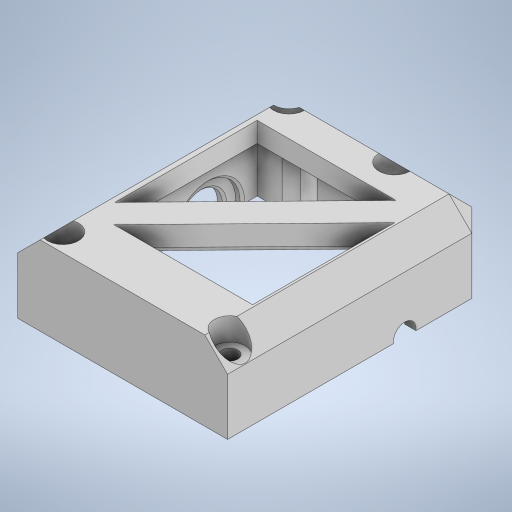
# Autodesk Inventor part: Arm_1_b
Saved by Autodesk Inventor 2023 (Build 270158000, 158)
## iProperties
Created: 2025-02-10
Part Number: Arm_1_b
Material: Generic
Document SubType Name: Modeling
Designer: Swoby
Density: 1 g/cm^3
Appearance: Default
Author: Swoby
Autodesk Inventor part; units mm, degrees
sketch "Sketch1" plane through (0, 0, 0) normal (0, 1, 0) x (-1, 0, 0)
  line L0 (0, 0) -> (3.1, 0)
  line L1 (0, 0) -> (0, -7.4)
  line L2 (0, -7.4) -> (1.5, -7.4)
  line L3 (1.5, -7.4) -> (1.5, -5)
  line L4 (1.5, -5) -> (3.1, -5)
  line L5 (3.1, -5) -> (3.1, 0)
  line L6 (0, -7.4) -> (0, -10.65)
  line L7 (0, -10.65) -> (-7.5, -10.65)
  line L8 (-7.5, -10.65) -> (-7.5, -17.75)
  line L9 (-7.5, -17.75) -> (-11.2, -17.75)
  line L10 (-11.2, -17.75) -> (-11.2, -10.65)
  line L11 (-11.2, -10.65) -> (-31.3, -10.65)
  line L12 (-31.3, -10.65) -> (-31.3, -19.75)
  line L13 (-31.3, -19.75) -> (-36.7, -19.75)
  line L14 (-36.7, -19.75) -> (-36.7, -10.65)
  line L15 (-36.7, -10.65) -> (-40.6, -10.65)
  line L16 (-40.6, -10.65) -> (-40.6, 30.95)
  line L17 (-40.6, 30.95) -> (-11.2, 30.95)
  line L18 (-11.2, 30.95) -> (-11.2, 38.05)
  line L19 (-11.2, 38.05) -> (-7.5, 38.05)
  line L20 (-7.5, 38.05) -> (-7.5, 30.95)
  line L21 (-7.5, 30.95) -> (0, 30.95)
  line L22 (0, 0) -> (0, 30.95)
  line L23 (3.1, 0) -> (3.1, 53.05)
  line L24 (-43.1, -19.75) -> (-43.1, 53.05)
  line L25 (3.1, -5) -> (3.1, -19.75)
  line L26 (3.1, -19.75) -> (-43.1047, -19.75)
  line L27 (-43.1, 53.05) -> (3.1, 53.05) construction
  line L28 (-43.1, 64.5353) -> (3.1, 64.5353) construction
  line L29 (3.1, 64.5353) -> (3.1, 93.4653) construction
  line L30 (3.1, 93.4653) -> (-43.1, 93.4653) construction
  line L31 (-43.1, 93.4653) -> (-43.1, 64.5353)
  line L32 (3.1, 53.05) -> (10.1, 60.05)
  line L33 (10.1, 60.05) -> (10.1, 95.4653)
  line L34 (10.1, 95.4653) -> (4.1, 95.4653)
  line L35 (4.1, 95.4653) -> (4.1, 62.5353)
  line L36 (4.1, 62.5353) -> (-5.3853, 53.05)
  line L37 (-20, 53.05) -> (-20, 57.2324) construction
  line L38 (-43.1, 64.5353) -> (-43.1, 93.4653)
  line L39 (-43.1, 53.05) -> (-50.1, 60.05)
  line L40 (-50.1, 60.05) -> (-50.1, 95.4653)
  line L41 (-50.1, 95.4653) -> (-44.1, 95.4653)
  line L42 (-44.1, 95.4653) -> (-44.1, 62.5353)
  line L43 (-44.1, 62.5353) -> (-34.6147, 53.05)
  line L44 (4.1, 62.5353) -> (10.1, 60.05) construction
  line L45 (-5.3853, 53.05) -> (-34.6147, 53.05)
  line L46 (-44.1, 79.0003) -> (-41.1, 79.0003)
  line L47 (-44.1, 81.3003) -> (-41.1, 81.3003)
  line L48 (-41.1, 81.3003) -> (-41.1, 79.0003)
  line L49 (-44.1, 81.3003) -> (-44.1, 79.0003)
  line L50 (-40.6, -2.5) -> (-40.6, 0)
  line L51 (-40.6, 0) -> (-43.1, 0)
  line L52 (-40.6, -2.5) -> (-43.1, -2.5)
  line L53 (-43.1, 0) -> (-43.1, -2.5)
  point P0 (1.55, 0)
  point P1 (-43.1, 65.1211)
  point P2 (-43.1, 94.8791)
  point P3 (3.1, 79.0003)
  dimension "d1" = 1.5
  dimension "d3" = 1.6
  dimension "d4" = 10
  dimension "d5" = 14.8
  dimension "d6" = 7.5
  dimension "d7" = 3.7
  dimension "d9" = 10.65
  dimension "d10" = 41.6
  dimension "d11" = 40.6
  dimension "d12" = 7.1
  dimension "d13" = 3.9
  dimension "d14" = 5.4
  dimension "d16" = 7.1
  dimension "d17" = 46.2
  dimension "d18" = 2
  dimension "d19" = 15
  dimension "d20" = 28.93
  dimension "d21" = 6
  dimension "d22" = 135
  dimension "d23" = 67.5
  dimension "d24" = 135
  dimension "d26" = 2
  dimension "d27" = 32.93
  dimension "d31" = 79.0003
  dimension "d33" = 1
  dimension "d34" = 3
  dimension "d35" = 2.3
  dimension "d70" = 5
  constraints: 108 end point, 24 perpendicular, 15 point on line, 7 collinear, 7 parallel, 7 vertical, 5 symmetric about line, 4 horizontal, 4 midpoint
  measures "d1" distance of L1.end L2.end
  measures "d3" distance of L3.end L4.end
  measures "d4" diameter of L4 L0
  measures "d5" diameter of L2 L0
  measures "d6" distance of L6.end L7.end
  measures "d7" distance of L8.end L9.end
  measures "d9" distance from line of L7 L0.start
  measures "d10" distance between parallel lines of L7 L21
  measures "d11" distance between parallel lines of L16 L22
  measures "d12" distance of L7.end L8.end
  measures "d13" distance of L14.end L15.end
  measures "d14" distance of L12.end L13.end
  measures "d16" distance of L19.end L20.end
  measures "d17" distance between parallel lines of L24 L23
  measures "d18" distance between parallel lines of L26 L9
  measures "d19" distance from line of L24.end L19
  measures "d20" distance of L28.end L29.end
  measures "d21" distance of L33.end L34.end
  measures "d22" angle of L23 L32
  measures "d23" angle of L32 L44
  measures "d24" angle of L32 L33
  measures "d26" distance from line of L30 L34.end
  measures "d27" distance from line of L34 L35.end
  measures "d31" vertical distance of point (3.1, 79) L0.start
  measures "d33" distance between parallel lines of L29 L35
  measures "d34" distance of L47.start L47.end
  measures "d35" distance of L47.end L46.end
  measures "d70" diameter of L52 L51
extrude "Extrusion1" add sketch "Sketch1" along normal mid plane 34 contours L22 L21 L20 L19 L18 L17 L16 L51 L24 L39 L40 L41 L42 L43 L45 L36 L35 L34 L33 L32 L23 L0 | L0 L5 L4 L3 L2 L1 | L2 L3 L4 L25 L26 L12 L11 L10 L9 L8 L7 L6 | L26 L24 L52 L16 L15 L14 | L24 L51 L16 L52
revolve "Revolution1" cut sketch "Sketch1" angle 360 about axis through (0, 0, 0) along (-1, 0, 0) contours L0 L5 L4 L3 L2 L1 | L24 L51 L16 L52
revolve "Revolution2" add sketch "Sketch1" angle 360 about axis through (44.1, 0, 79.0003) along (-1, 0, 0) contours L42 L47 L31 L46 | L31 L47 L48 L46
sketch "Sketch2" plane through (-4.1, -17, 62.5353) normal (1, 0, 0) x (0, 0, -1)
  line L0 (-32.93, 34) -> (0, 0) construction
  line L1 (0, 34) -> (-32.93, 0) construction
  circle A0 centre (-16.465, 17) radius 3.4
  line L2 (-16.465, 17) -> (-5.3446, 17) construction
  line L3 (-16.465, 17) -> (-3.5603, 29.9047) construction
  line L4 (-16.465, 17) -> (-3.5603, 4.0953) construction
  circle A1 centre (-3.5603, 29.9047) radius 0.5
  arc A2 (-1.9362, 28.7375) -> (-2.1461, 31.3189) centre (-3.5603, 29.9047) ccw
  arc A3 (-2.1461, 2.6811) -> (-1.9362, 5.2625) centre (-3.5603, 4.0953) ccw
  circle A4 centre (-3.5603, 4.0953) radius 0.5
  line L5 (-11.8688, 21.5962) -> (-9.0757, 18.8031) construction
  line L6 (-11.8688, 12.4038) -> (-9.0757, 15.1969) construction
  line L7 (-9.0757, 15.1969) -> (-1.9362, 5.2625)
  line L8 (-9.0757, 18.8031) -> (-1.9362, 28.7375)
  line L9 (-3.5603, 29.9047) -> (-2.1461, 31.3189) construction
  line L10 (-3.5603, 4.0953) -> (-2.1461, 2.6811) construction
  line L11 (-3.5603, 29.9047) -> (-2.1461, 31.3189) construction
  arc A5 (-9.0757, 18.8031) -> (-9.0757, 15.1969) centre (-6.5668, 17) ccw
  arc A6 (-28.2025, 31.5288) -> (-30.7839, 31.3189) centre (-29.3697, 29.9047) ccw
  line L12 (-18.2681, 24.3893) -> (-28.2025, 31.5288)
  arc A7 (-18.2681, 24.3893) -> (-14.6619, 24.3893) centre (-16.465, 26.8982) ccw
  line L13 (-14.6619, 24.3893) -> (-4.7275, 31.5288)
  arc A8 (-2.1461, 31.3189) -> (-4.7275, 31.5288) centre (-3.5603, 29.9047) ccw
  circle A9 centre (-3.5603, 29.9047) radius 0.5
  circle A10 centre (-29.3697, 29.9047) radius 0.5
  arc A11 (-30.9938, 5.2625) -> (-30.7839, 2.6811) centre (-29.3697, 4.0953) ccw
  line L14 (-23.8543, 15.1969) -> (-30.9938, 5.2625)
  arc A12 (-23.8543, 15.1969) -> (-23.8543, 18.8031) centre (-26.3632, 17) ccw
  line L15 (-23.8543, 18.8031) -> (-30.9938, 28.7375)
  arc A13 (-30.7839, 31.3189) -> (-30.9938, 28.7375) centre (-29.3697, 29.9047) ccw
  circle A14 centre (-29.3697, 29.9047) radius 0.5
  circle A15 centre (-29.3697, 4.0953) radius 0.5
  arc A16 (-4.7275, 2.4712) -> (-2.1461, 2.6811) centre (-3.5603, 4.0953) ccw
  line L16 (-14.6619, 9.6107) -> (-4.7275, 2.4712)
  arc A17 (-14.6619, 9.6107) -> (-18.2681, 9.6107) centre (-16.465, 7.1018) ccw
  line L17 (-18.2681, 9.6107) -> (-28.2025, 2.4712)
  arc A18 (-30.7839, 2.6811) -> (-28.2025, 2.4712) centre (-29.3697, 4.0953) ccw
  circle A19 centre (-29.3697, 4.0953) radius 0.5
  circle A20 centre (-3.5603, 4.0953) radius 0.5
  point P0 (62.5353, 17)
  point P1 (-2.1461, 31.3189)
  point P2 (-30.7839, 31.3189)
  point P3 (-30.7839, 2.6811)
  point P4 (-2.1461, 2.6811)
  dimension "d38" = 6.8
  dimension "d39" = 45
  dimension "d40" = 1
  dimension "d41" = 4
  dimension "d42" = 18.25
  dimension "d43" = 18.25
  dimension "d44" = 4
  dimension "d45" = 1
  dimension "d46" = 3.95
  dimension "d47" = 6.5
  dimension "d48" = 3.95
  dimension "d49" = 6.5
  dimension "d52" = 360
  constraints: 36 end point, 24 point on circle, 21 centre point, 10 coincident, 3 point on line, 3 tangent, 2 midpoint, 1 collinear, 1 horizontal, 1 perpendicular, 73 other
  measures "d38" diameter of A0
  measures "d39" angle of L2 L3
  measures "d40" diameter of A1
  measures "d41" diameter of A2
  measures "d42" distance of L3.end point (-16.465, 17)
  measures "d43" distance of L2.start L4.end
  measures "d44" diameter of A3
  measures "d45" diameter of A4
  measures "d46" distance of L5.start L5.end
  measures "d47" distance between parallel lines of L4 L5
  measures "d48" distance of L6.start L6.end
  measures "d49" distance between parallel lines of L3 L6
extrude "Extrusion2" cut sketch "Sketch2" against normal through all contours A0 | A1 | A4 | A10 | A15
extrude "Extrusion3" cut sketch "Sketch2" against normal blind 4
sketch "Sketch3" plane through (0, 17, 0) normal (0, 1, 0) x (1, 0, 0)
  line L0 (43.1, -53.05) -> (43.1, 19.75) projected
  line L1 (43.1, 19.75) -> (36.7, 19.75) projected
  line L2 (36.7, 19.75) -> (36.7, 10.65) projected
  line L3 (36.7, 10.65) -> (40.6, 10.65) projected
  line L4 (40.6, 10.65) -> (40.6, -30.95) projected
  line L5 (40.6, -30.95) -> (11.2, -30.95) projected
  line L6 (11.2, -30.95) -> (11.2, -38.05) projected
  line L7 (11.2, -38.05) -> (7.5, -38.05) projected
  line L8 (7.5, -38.05) -> (7.5, -30.95) projected
  line L9 (7.5, -30.95) -> (0, -30.95) projected
  line L10 (0, -30.95) -> (0, 10.65) projected
  line L11 (0, 10.65) -> (7.5, 10.65) projected
  line L12 (7.5, 10.65) -> (7.5, 17.75) projected
  line L13 (7.5, 17.75) -> (11.2, 17.75) projected
  line L14 (11.2, 17.75) -> (11.2, 10.65) projected
  line L15 (11.2, 10.65) -> (31.3, 10.65) projected
  line L16 (31.3, 10.65) -> (31.3, 19.75) projected
  line L17 (31.3, 19.75) -> (-3.1, 19.75) projected
  line L18 (-3.1, 19.75) -> (-3.1, -53.05) projected
  line L19 (-3.1, -53.05) -> (-10.1, -60.05) projected
  line L20 (-10.1, -60.05) -> (-10.1, -95.4653) projected
  line L21 (-10.1, -95.4653) -> (-4.1, -95.4653) projected
  line L22 (-4.1, -95.4653) -> (-4.1, -62.5353) projected
  line L23 (-4.1, -62.5353) -> (5.3853, -53.05) projected
  line L24 (5.3853, -53.05) -> (34.6147, -53.05) projected
  line L25 (34.6147, -53.05) -> (44.1, -62.5353) projected
  line L26 (44.1, -62.5353) -> (44.1, -95.4653) projected
  line L27 (44.1, -95.4653) -> (50.1, -95.4653) projected
  line L28 (50.1, -95.4653) -> (50.1, -60.05) projected
  line L29 (50.1, -60.05) -> (43.1, -53.05) projected
  line L30 (31.3, 19.75) -> (36.7, 19.75)
  point P0 (0, 0)
  constraints: 2 end point, 1 collinear
extrude "Extrusion4" add sketch "Sketch3" against normal blind 6.4 contours L2 L3 L4 L5 L6 L7 L8 L9 L10 L11 L12 L13 L14 L15 L16 L30
mirror "Mirror1" about plane through (0, 0, 0) normal (0, 1, 0) of "Extrusion4"
chamfer "Chamfer1" distance 3 angle 45 4 edges at (47.1, -17, 95.4653) (47.1, 17, 95.4653) (-7.1, -17, 95.4653) (-7.1, 17, 95.4653)
chamfer "Chamfer2" distance 5 angle 45 10 edges at (-3.1, -17, 16.65) (43.1, -17, 16.65) (43.1, 0, -19.75) (20, -17, -19.75) (43.1, 17, 16.65) (20, 17, -19.75) (-3.1, 17, 16.65) (-3.1, 0, -19.75) (20, -17, 53.05) (20, 17, 53.05)
chamfer "Chamfer3" distance 2 angle 45 34 edges at (-6.6, -17, 56.55) (0.6426, -17, 57.7926) (-10.1, -17, 76.2576) (-4.1, -17, 77.5003) (39.3574, -17, 57.7926) (46.6, -17, 56.55) (50.1, -17, 76.2576) (44.1, -17, 77.5003) (50.1, 0, 60.05) (-10.1, 0, 60.05) (-6.6, 17, 56.55) (-10.1, 17, 76.2576) (-10.1, 0, 95.4653) (-10.1, 15.5, 93.9653) (-10.1, -15.5, 93.9653) (-4.1, -15.5, 93.9653) (-4.1, 0, 95.4653) (-4.1, 15.5, 93.9653) (-4.1, 17, 77.5003) (0.6426, 17, 57.7926) (39.3574, 17, 57.7926) (46.6, 17, 56.55) (44.1, 17, 77.5003) (50.1, 17, 76.2576) (44.1, 15.5, 93.9653) (44.1, 0, 95.4653) (44.1, -15.5, 93.9653) (50.1, -15.5, 93.9653) (50.1, 0, 95.4653) (50.1, 15.5, 93.9653) (20, -12, 53.05) (20, -17, 48.05) (20, 12, 53.05) (20, 17, 48.05)
sketch "Sketch4" plane through (0, 17, 0) normal (0, 1, 0) x (1, 0, 0)
  line L0 (11.2, 10.65) -> (31.3, 10.65) projected
  line L1 (11.2, 17.75) -> (11.2, 10.65) projected
  line L2 (7.5, 17.75) -> (11.2, 17.75) projected
  line L3 (7.5, 10.65) -> (7.5, 17.75) projected
  line L4 (0, 10.65) -> (7.5, 10.65) projected
  line L5 (0, -30.95) -> (0, 10.65) projected
  line L6 (7.5, -30.95) -> (0, -30.95) projected
  line L7 (7.5, -38.05) -> (7.5, -30.95) projected
  line L8 (11.2, -38.05) -> (7.5, -38.05) projected
  line L9 (11.2, -30.95) -> (11.2, -38.05) projected
  line L10 (40.6, -30.95) -> (11.2, -30.95) projected
  line L11 (40.6, 10.65) -> (40.6, -30.95) projected
  line L12 (36.7, 10.65) -> (40.6, 10.65) projected
  line L13 (36.7, 19.75) -> (36.7, 10.65) projected
  line L14 (31.3, 19.75) -> (36.7, 19.75) projected
  line L15 (31.3, 10.65) -> (31.3, 19.75) projected
  line L16 (33.4802, 7.65) -> (3, 7.65)
  line L17 (7.1198, -27.95) -> (37.6, -27.95)
  line L18 (40.6, 10.65) -> (0, -30.95) construction
  line L19 (33.4802, 7.65) -> (3, -23.5809)
  line L20 (7.1198, -27.95) -> (37.6, 3.2809)
  line L21 (37.6, -27.95) -> (37.6, 3.2809)
  line L22 (37.6, 7.5761) -> (37.6, 7.65)
  line L23 (3, 7.65) -> (3, -23.5809)
  line L24 (3, -27.8761) -> (3, -27.95)
  point P0 (0, 0)
  point P1 (20.3, -10.15)
  dimension "d72" = 3
  dimension "d74" = 3
  dimension "d75" = 3
  dimension "d76" = 3
  dimension "d77" = 3
  dimension "d78" = 3
  constraints: 18 end point, 7 parallel, 2 perpendicular, 2 point on line, 1 horizontal, 1 midpoint
  measures "d72" distance between parallel lines of L10 L17
  measures "d74" distance between parallel lines of L0 L16
  measures "d75" distance from line of point (20.3, -10.15) L19
  measures "d76" distance between parallel lines of L20 L18
  measures "d77" distance between parallel lines of L5 L23
  measures "d78" distance between parallel lines of L11 L21
extrude "Extrusion5" cut sketch "Sketch4" against normal through all contours L19 L23 L16 | L20 L21 L17
chamfer "Chamfer4" distance 2 angle 45 16 edges at (18.2401, -10.6, 7.9655) (22.3599, -10.6, 12.3345) (18.2401, 10.6, 7.9655) (22.3599, 10.6, 12.3345) (18.2401, -10.6, -7.65) (3, -10.6, 7.9655) (3, 10.6, 7.9655) (18.2401, 10.6, -7.65) (37.6, 10.6, 12.3345) (22.3599, 10.6, 27.95) (22.3599, -10.6, 27.95) (37.6, -10.6, 12.3345) (7.5, 0, 30.95) (11.2, 0, 30.95) (7.5, 0, -10.65) (11.2, 0, -10.65)
ref_plane "Work Plane2" through (0, -0.4, 0) normal (0, -1, 0) x (1, 0, 0)
ref_plane "Work Plane3" through (40.6, -10.6, 38.95) normal (0, 0, -1) x (-1, 0, 0)
sketch "Sketch5" plane through (0, -0.4, 0) normal (0, -1, 0) x (1, 0, 0)
  line L0 (62.14, 38.95) -> (-22.14, 38.95) projected
  line L1 (43.1, -14.75) -> (43.1, 53.05) projected
  line L2 (43.1, -14.75) -> (38.1, -19.75) projected
  line L3 (1.9, -19.75) -> (38.1, -19.75) projected
  line L4 (36.7, -19.75) -> (36.7, -10.65) projected
  line L5 (36.7, -10.65) -> (40.6, -10.65) projected
  line L6 (40.6, -10.65) -> (40.6, 30.95) projected
  line L7 (40.6, 30.95) -> (13.2, 30.95) projected
  line L8 (13.2, 30.95) -> (11.2, 32.95) projected
  line L9 (11.2, 32.95) -> (11.2, 38.05) projected
  line L10 (11.2, 38.05) -> (7.5, 38.05) projected
  line L11 (7.5, 38.05) -> (7.5, 32.95) projected
  line L12 (7.5, 32.95) -> (5.5, 30.95) projected
  line L13 (5.5, 30.95) -> (0, 30.95) projected
  line L14 (0, 30.95) -> (0, -10.65) projected
  line L15 (0, -10.65) -> (5.5, -10.65) projected
  line L16 (5.5, -10.65) -> (7.5, -12.65) projected
  line L17 (7.5, -12.65) -> (7.5, -17.75) projected
  line L18 (7.5, -17.75) -> (11.2, -17.75) projected
  line L19 (11.2, -17.75) -> (11.2, -12.65) projected
  line L20 (1, 28.4936) -> (38.2267, -9.65) projected
  line L21 (1, -9.65) -> (1, 28.4936) projected
  line L22 (38.2267, -9.65) -> (1, -9.65) projected
  line L23 (11.2, -12.65) -> (13.2, -10.65) projected
  line L24 (11.2, -17.75) -> (11.2, -12.65) projected
  line L25 (7.5, -17.75) -> (11.2, -17.75) projected
  line L26 (7.5, -12.65) -> (7.5, -17.75) projected
  line L27 (5.5, -10.65) -> (7.5, -12.65) projected
  line L28 (0, -10.65) -> (5.5, -10.65) projected
  line L29 (0, 30.95) -> (0, -10.65) projected
  line L30 (5.5, 30.95) -> (0, 30.95) projected
  line L31 (7.5, 32.95) -> (5.5, 30.95) projected
  line L32 (7.5, 38.05) -> (7.5, 32.95) projected
  line L33 (11.2, 38.05) -> (7.5, 38.05) projected
  line L34 (11.2, 32.95) -> (11.2, 38.05) projected
  line L35 (13.2, 30.95) -> (11.2, 32.95) projected
  line L36 (40.6, 30.95) -> (13.2, 30.95) projected
  line L37 (40.6, -10.65) -> (40.6, 30.95) projected
  line L38 (36.7, -10.65) -> (40.6, -10.65) projected
  line L39 (36.7, -19.75) -> (36.7, -10.65) projected
  line L40 (31.3, -19.75) -> (36.7, -19.75) projected
  line L41 (31.3, -10.65) -> (31.3, -19.75) projected
  line L42 (13.2, -10.65) -> (31.3, -10.65) projected
  line L43 (39.6, -8.1936) -> (2.3733, 29.95) projected
  line L44 (39.6, 29.95) -> (39.6, -8.1936) projected
  line L45 (2.3733, 29.95) -> (39.6, 29.95) projected
  line L46 (1.9, -19.75) -> (-3.1, -14.75) projected
  line L47 (-3.1, 53.05) -> (-3.1, -14.75) projected
  circle A0 centre (26.1, -14.75) radius 2.15
  line L48 (36.7, -14.75) -> (43.1, -14.75) construction
  line L49 (26.1, -14.75) -> (26.1, -19.75) construction
  circle A1 centre (2.9, -14.75) radius 2.15
  circle A2 centre (39.6, 34.95) radius 2.15
  circle A3 centre (2.9, 34.95) radius 2.15
  circle A4 centre (2.9, -14.75) radius 1.75
  circle A5 centre (26.1, -14.75) radius 1.75
  circle A6 centre (39.6, 34.95) radius 1.75
  circle A7 centre (2.9, 34.95) radius 1.75
  circle A8 centre (26.1, -14.75) radius 3.4
  circle A9 centre (2.9, -14.75) radius 3.4
  circle A10 centre (2.9, 34.95) radius 3.4
  circle A11 centre (39.6, 34.95) radius 3.4
  point P0 (0, 0)
  dimension "d86" = 4.3
  dimension "d87" = 5
  dimension "d89" = 4.3
  dimension "d90" = 6
  dimension "d91" = 4.3
  dimension "d92" = 4
  dimension "d93" = 8
  dimension "d94" = 4.3
  dimension "d95" = 4
  dimension "d96" = 6
  dimension "d101" = 3.5
  dimension "d102" = 3.5
  dimension "d103" = 3.5
  dimension "d104" = 3.5
  dimension "d105" = 6.8
  dimension "d106" = 6.8
  dimension "d107" = 6.8
  dimension "d108" = 6.8
  dimension "d111" = 17
  constraints: 12 centre point, 8 coincident, 6 point on line, 4 end point, 1 perpendicular, 1 vertical
  measures "d86" diameter of A0
  measures "d87" distance between parallel lines of L3 L48
  measures "d89" diameter of A1
  measures "d90" distance from line of L47 A1.centre
  measures "d91" diameter of A2
  measures "d92" distance from line of L0 A2.centre
  measures "d93" distance between parallel lines of L0 L36
  measures "d94" diameter of A3
  measures "d95" distance from line of L0 A3.centre
  measures "d96" distance from line of L47 A3.centre
  measures "d101" diameter of A4
  measures "d102" diameter of A5
  measures "d103" diameter of A6
  measures "d104" diameter of A7
  measures "d105" diameter of A8
  measures "d106" diameter of A9
  measures "d107" diameter of A10
  measures "d108" diameter of A11
  measures "d111" distance between parallel lines of L49 L1
extrude "Extrusion6" cut sketch "Sketch5" along normal blind 18 contours A0 | A1 | A2 | A3 | A4 | A5 | A6 | A7
sketch "Sketch6" plane through (-10.1, -15, 62.05) normal (-1, 0, 0) x (0, 0, 1)
  line L0 (-9, 27) -> (-12, 30) construction
  line L1 (-11.1716, 32) -> (-12, 30) construction
  line L2 (-11.1716, 32) -> (-76.8, 32) construction
  line L3 (-76.8, 32) -> (-76.8, 27) construction
  line L4 (-76.8, 27) -> (-9, 27) construction
  line L5 (-81.8, 27) -> (-76.8, 32) construction
  line L6 (-76.8, 27) -> (-81.8, 27) construction
  line L7 (-76.8, 32) -> (-76.8, 27) construction
  line L8 (-76.8, 27) -> (-81.8, 27) construction
  line L9 (-81.8, 27) -> (-81.8, 3) construction
  line L10 (-81.8, 3) -> (-76.8, 3) construction
  line L11 (-76.8, 3) -> (-76.8, 27) construction
  line L12 (-9, 3) -> (-76.8, 3) construction
  line L13 (-9, 3) -> (-9, 27) construction
  line L14 (-76.8, 27) -> (-9, 27) construction
  line L15 (-76.8, 3) -> (-76.8, 27) construction
  circle A0 centre (-62.05, 15) radius 5 construction
  line L16 (56.4583, 14.6) -> (-104.8431, 14.6) construction
  line L17 (-23.1, -8.8) -> (-23.1, 38.8) construction
  line L18 (-23.1, 14.6) -> (-81.8, 14.6)
  line L19 (-81.8, 14.6) -> (-81.8, 27)
  line L20 (-81.8, 27) -> (-76.8, 32)
  line L21 (-76.8, 32) -> (-23.1, 32)
  line L22 (-23.1, 32) -> (-23.1, 14.6)
  line L23 (-76.8, -2) -> (-11.1716, -2) projected
  line L24 (-11.1716, -2) -> (-1.1716, -2) projected
  line L25 (-1.1716, -2) -> (30.4153, -2) projected
  line L26 (30.4153, -2) -> (33.4153, 1) projected
  line L27 (33.4153, 1) -> (33.4153, 29) projected
  line L28 (33.4153, 29) -> (30.4153, 32) projected
  line L29 (30.4153, 32) -> (-1.1716, 32) projected
  line L30 (-81.8, 14.6) -> (-81.8, 3)
  line L31 (-81.8, 3) -> (-76.8, -2)
  line L32 (-76.8, -2) -> (30.4153, -2)
  line L33 (30.4153, -2) -> (33.4153, 1)
  line L34 (33.4153, 29) -> (33.4153, 1)
  line L35 (33.4153, 29) -> (30.4153, 32)
  line L36 (30.4153, 32) -> (-23.1, 32)
  constraints: 24 end point, 7 collinear, 6 point on line, 2 perpendicular
extrude "Extrusion7" cut sketch "Sketch6" against normal through all contours L22 L36 L29 L28 L27 L26 L25 L24 L23 L31 L30 L18
extrude "Extrusion8" cut sketch "Sketch5" against normal through all contours A4 | A5 | A6 | A7
ref_plane "Work Plane4" through (-3.1, 12, 9.0538) normal (0, -1, 0) x (0, 0, 1)
extrude "Extrusion9" cut sketch "Sketch5" against normal up to surface (5 mm away) from surface at -12.4 contours A0 | A1 | A2 | A3 | A4 | A5 | A6 | A7 | A8 | A9 | A10 | A11
chamfer "Chamfer5" distance 0.5 angle 45 2 edges at (0, 7.4, 0) (-1.5, 5, 0)
equation "\"d16\" = d12"
equation "\"d23\" = 0.5 * d24"
equation "\"d27\" = d20 + 2 * d26"
equation "\"d43\" = d42"
equation "\"d49\" = d47"
equation "\"d72\" = d71"
equation "\"d74\" = d71"
equation "\"d76\" = d71"
equation "\"d77\" = d75"
equation "\"d78\" = d75"
equation "\"d92\" = 0.5 * d93"
equation "\"d95\" = d92"
equation "\"d96\" = d90"
equation "\"d73\" = d71"
equation "\"d71\" = 3"
body "Solid1"
